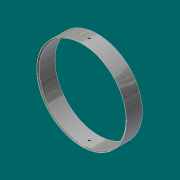
# Autodesk Inventor part: A1-19027-300-01 32in pipe
Saved by Autodesk Inventor 2017.3 (Build 213257000, 257)
## iProperties
Created: 2019-09-12
Part Number: A1-19027-300-01 32in pipe
Material: Steel, Mild
Document SubType Name: Modeling
Designer: GVD
Density: 7.85 g/cm^3
Appearance: Steel
Mass: 36399.6 g
Surface Area: 8061.28 cm^2
Volume: 4636.89 cm^3
Description: 32" XS x 6 1/32" PIPE, API 5L Gr.B
Author: GVD
Autodesk Inventor part; units mm, degrees
ref_plane "YZ Plane" through (0, 0, 0) normal (1, 0, 0) x (0, 1, 0)
ref_plane "XY Plane" through (0, 0, 0) normal (0, 0, 1) x (1, 0, 0)
sketch "Sketch1" plane through (0, 0, 0) normal (0, 0, 1) x (1, 0, 0)
  circle A0 centre (0, 0) radius 406.4
  circle A1 centre (0, 0) radius 393.7
  dimension "d0" = 812.8
  dimension "d1" = 787.4
  constraints: 2 centre point, 2 coincident
  measures "d0" diameter of A0
  measures "d1" diameter of A1
extrude "Extrusion1" add sketch "Sketch1" along normal blind 153.4
chamfer "Chamfer1" distance 11.1125 angle 37.5 1 edges at (-406.4, 0, 0) measured on face at (-405.9, 0, 0)
chamfer "Chamfer2" distance 11.1125 angle 40 1 edges at (-393.7, 0, 153.4) measured on face at (-394.2, 0, 153.4)
ref_plane "Work Plane1" through (0, 406.4, 0) normal (0, 1, 0) x (-1, 0, 0)
sketch "Sketch2" plane through (0, 406.4, 0) normal (0, 1, 0) x (-1, 0, 0)
  point P0 (0, 0)
  point P1 (0, 57.9438)
  dimension "d10" = 57.9438
  constraints: 1 vertical alignment
  measures "d10" distance of point (0, 0) point (0, 57.944)
hole "Hole1" at (0, 406.4, 57.9438) direction (0, -1, 0) diameter 22.6314 depth 23.114 tip angle 118 taper from width 23.6614 to width 22.7838 over 14.0462 thread size "3/4" designation "3/4 - 14 NPT" standard "NPT"
pattern_circular "Circular Pattern1" count 2 over 360 about axis through (0, 0, -10) along (0, 0, 1) of "Hole1"
equation "\"d7\" = d4"
equation "\"d4\" = 11.1125"
body "Solid1"
